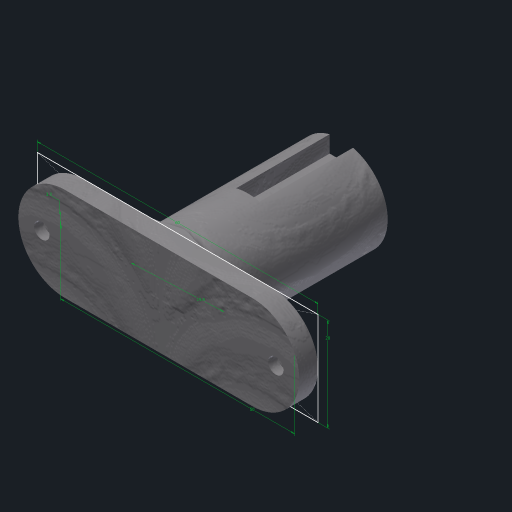
# Autodesk Inventor part: GIRO_1
Saved by Autodesk Inventor 2024.3 (Build 283343000, 343)
## iProperties
Created: 2024-07-12
Part Number: GIRO_1
Material: Steel, Mild, Welded
Document SubType Name: Modeling
Designer: Niler
Density: 7.85 g/cm^3
Appearance: Weld - Steel Mild
Author: Niler
Autodesk Inventor part; units mm, degrees
ref_plane "YZ Plane" through (0, 0, 0) normal (1, 0, 0) x (0, 1, 0)
ref_plane "XZ Plane" through (0, 0, 0) normal (0, 1, 0) x (-1, 0, 0)
ref_plane "XY Plane" through (0, 0, 0) normal (0, 0, 1) x (1, 0, 0)
sketch "Sketch1" plane through (0, 0, 0) normal (0, 0, 1) x (1, 0, 0)
  line L0 (-30, -10) -> (30, -10)
  line L1 (30, -10) -> (30, 10)
  line L2 (30, 10) -> (-30, 10)
  line L3 (-30, 10) -> (-30, -10)
  line L4 (-30, -10) -> (30, 10) construction
  line L5 (30, -10) -> (-30, 10) construction
  circle A0 centre (0, 0) radius 9.9
  circle A1 centre (-25, 0) radius 1.65
  circle A2 centre (25, 0) radius 1.65
  line L6 (-25, 0) -> (25, 0) construction
  point P0 (-30, 0)
  dimension "d0" = 60
  dimension "d1" = 19.8
  dimension "d2" = 20
  dimension "d3" = 50
  dimension "d4" = 3.3
  constraints: 14 end point, 4 midpoint, 3 centre point, 2 horizontal, 2 horizontal alignment, 2 parallel, 1 coincident, 1 equal radius, 1 perpendicular
  measures "d0" distance of L2.end L1.end
  measures "d1" diameter of A0
  measures "d2" distance of L0.end L1.end
  measures "d3" distance of L6.end L6.start
  measures "d4" diameter of A1
extrude "Extrusion1" add sketch "Sketch1" along normal blind 4 contours L3 L2 L1 L0 | A0
extrude "Extrusion2" add sketch "Sketch1" against normal blind 35 contours A0
fillet "Fillet1" radius 2 1 edges at (-9.9, 0, 0)
fillet "Fillet2" radius 10 4 edges at (30, 10, 2) (30, -10, 2) (-30, 10, 2) (-30, -10, 2)
sketch "Sketch2" plane through (0, 0, -35) normal (0, 0, -1) x (-1, 0, 0)
  circle A0 centre (0, 0) radius 9.9 projected
  line L0 (-2.5, 0) -> (2.5, 0)
  line L1 (2.5, 0) -> (2.5, 12)
  line L2 (2.5, 12) -> (-2.5, 12)
  line L3 (-2.5, 12) -> (-2.5, 0)
  line L4 (-2.5, 6) -> (2.5, 6)
  point P0 (0, 12)
  point P1 (2.5, 9.5791)
  point P2 (-2.5, 9.5791)
  dimension "d11" = 12
  dimension "d12" = 5
  dimension "d13" = 6
  constraints: 10 end point, 4 midpoint, 2 parallel, 2 perpendicular, 1 coincident, 1 horizontal, 1 vertical alignment
  measures "d11" distance from line of point (0, 0) L2
  measures "d12" distance between parallel lines of L1 L3
  measures "d13" distance between parallel lines of L0 L4
extrude "Extrusion3" cut sketch "Sketch2" against normal blind 20 contours L1 L4 L3 A0
sketch "Sketch3" plane through (0, 0, 0) normal (0, 0, -1) x (-1, 0, 0)
  arc A0 (-20, 10) -> (-20, -10) centre (-20, 0) ccw projected
  line L0 (-6.4506, -10) -> (-20, -10) projected
  arc A1 (-6.4506, 10) -> (-6.4506, -10) centre (0, 0) ccw projected
  line L1 (-20, 10) -> (-6.4506, 10) projected
  circle A2 centre (-25, 0) radius 1.65 projected
  line L2 (-28.3486, 0) -> (-26.6743, 2.9)
  line L3 (-26.6743, 2.9) -> (-23.3257, 2.9)
  line L4 (-23.3257, 2.9) -> (-21.6514, 0)
  line L5 (-21.6514, 0) -> (-23.3257, -2.9)
  line L6 (-23.3257, -2.9) -> (-26.6743, -2.9)
  line L7 (-26.6743, -2.9) -> (-28.3486, 0)
  circle A3 centre (25, 0) radius 1.65 projected
  line L8 (23.3257, 2.9) -> (26.6743, 2.9)
  line L9 (26.6743, 2.9) -> (28.3486, 0)
  line L10 (28.3486, 0) -> (26.6743, -2.9)
  line L11 (26.6743, -2.9) -> (23.3257, -2.9)
  line L12 (23.3257, -2.9) -> (21.6514, 0)
  line L13 (21.6514, 0) -> (23.3257, 2.9)
  point P0 (-25, 2.9)
  dimension "d16" = 5.8
  dimension "d17" = 5.8
  constraints: 24 end point, 2 coincident, 2 horizontal alignment, 1 midpoint, 26 other
  measures "d16" distance from line of L6 point (-25, 2.9)
  measures "d17" distance between parallel lines of L11 L8
extrude "Extrusion4" cut sketch "Sketch3" against normal blind 2 contours L2 L3 L4 L5 L6 L7 | L8 L9 L10 L11 L12 L13
body "Solid1"
